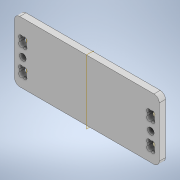
# Autodesk Inventor part: side_side
Saved by Autodesk Inventor 2020 (Build 240168000, 168)
## iProperties
Created: 2020-01-09
Part Number: side_side
Material: Generic
Document SubType Name: Modeling
Designer: erwin
Density: 1 g/cm^3
Appearance: Default
Author: erwin
Autodesk Inventor part; units mm, degrees
ref_plane "YZ Plane" through (0, 0, 0) normal (1, 0, 0) x (0, 1, 0)
ref_plane "XZ Plane" through (0, 0, 0) normal (0, 1, 0) x (-1, 0, 0)
ref_plane "XY Plane" through (0, 0, 0) normal (0, 0, 1) x (1, 0, 0)
ref_plane "Work Plane1" through (0, 0, 0) normal (0, 0, 1) x (1, 0, 0)
ref_plane "Work Plane2" through (0, 0, 0) normal (0, 0, 1) x (1, 0, 0)
sketch "Sketch2" plane through (0, 0, 0) normal (0, 0, 1) x (1, 0, 0)
  line L0 (-3.6, 30) -> (-3.6, 22) projected
  line L1 (70, 0.0472) -> (70, -3.6) projected
  line L2 (73.6, 0.0472) -> (73.6, -3.6) projected
  line L3 (-3.6, 30) -> (73.6, 30)
  line L4 (73.6, 30) -> (73.6, -3.6)
  line L5 (73.6, -3.6) -> (-3.6, -3.6)
  line L6 (-3.6, -3.6) -> (-3.6, 30)
  line L7 (70, 7) -> (70, 2) projected
  line L8 (73.6, 7) -> (73.6, 2) projected
  line L9 (70, 22) -> (70, 17) projected
  line L10 (73.6, 22) -> (73.6, 17) projected
  line L11 (0, 22) -> (-3.6, 22) projected
  line L12 (-3.6, 17) -> (-3.6, 22) projected
  line L13 (-3.6, 17) -> (0, 17) projected
  line L14 (0, 17) -> (0, 22) projected
  line L15 (-3.6, 2) -> (0, 2) projected
  line L16 (0, 2) -> (0, 7) projected
  line L17 (0, 7) -> (-3.6, 7) projected
  line L18 (-3.6, 2) -> (-3.6, 7) projected
  line L19 (70, 2) -> (73.6, 2) projected
  line L20 (70, 7) -> (73.6, 7) projected
  line L21 (70, 17) -> (73.6, 17) projected
  line L22 (70, 22) -> (73.6, 22) projected
  line L23 (70, 0.0472) -> (73.6, 0.0472) projected
  line L24 (70, -3.6) -> (73.6, -3.6) projected
  point P0 (0, 0)
  point P1 (-3.6, 22)
  constraints: 8 end point, 2 parallel, 1 horizontal, 1 perpendicular
extrude "Extrusion1" add sketch "Sketch2" along normal blind 3.6 contours L3 L4 L22 L9 L21 L20 L7 L19 L23 L1 L5 L6 L15 L16 L17 L13 L14 L11 L0 | L1 L23 L2 L5
ref_plane "Work Plane6" through (35, -3.6, 0) normal (1, 0, 0) x (0, 0, -1)
sketch "Sketch3" plane through (0, 0, 3.6) normal (0, 0, 1) x (1, 0, 0)
  line L0 (-3.6, 30) -> (-3.6, 22) projected
  line L1 (73.6, -3.6) -> (73.6, 2) projected
  line L2 (73.6, 30) -> (-3.6, 30) projected
  line L3 (-3.6, 30) -> (-3.6, -3.6) projected
  line L4 (-3.6, 30) -> (-3.6, 30)
  line L5 (-6.6, 27) -> (-6.6, -0.6)
  line L6 (-3.6, -3.6) -> (-3.6, -3.6)
  line L7 (-3.6, -3.6) -> (-3.6, 30)
  arc A0 (-3.6, 30) -> (-6.6, 27) centre (-3.6, 27) ccw
  arc A1 (-6.6, -0.6) -> (-3.6, -3.6) centre (-3.6, -0.6) ccw
  line L8 (-3.6, -3.6) -> (73.6, -3.6) projected
  line L9 (70, 2) -> (70, 7) projected
  line L10 (70, 7) -> (73.6, 7) projected
  line L11 (73.6, 7) -> (73.6, 17) projected
  line L12 (73.6, 17) -> (70, 17) projected
  line L13 (70, 17) -> (70, 22) projected
  line L14 (70, 22) -> (73.6, 22) projected
  line L15 (73.6, 22) -> (73.6, 30) projected
  line L16 (-3.6, 22) -> (0, 22) projected
  line L17 (0, 22) -> (0, 17) projected
  line L18 (0, 17) -> (-3.6, 17) projected
  line L19 (-3.6, 17) -> (-3.6, 7) projected
  line L20 (-3.6, 7) -> (0, 7) projected
  line L21 (0, 7) -> (0, 2) projected
  line L22 (0, 2) -> (-3.6, 2) projected
  line L23 (-3.6, 2) -> (-3.6, -3.6) projected
  line L24 (73.6, 2) -> (70, 2) projected
  point P0 (0, 0)
  point P1 (-6.6, -3.6)
  point P2 (-3.6, 22)
  point P3 (-3.6, 30)
  point P4 (-3.6, 30)
  dimension "d2" = 3
  dimension "d3" = 3
  constraints: 8 end point, 4 point on circle, 4 tangent, 2 centre point, 2 parallel, 2 point on line, 1 equal radius, 1 horizontal, 1 perpendicular
  measures "d2" distance of L3.end point (-6.6, -3.6)
  measures "d3" radius of A0
extrude "Extrusion2" add sketch "Sketch3" against normal blind 3.6 contours L0 L3 A1 L5 A0
sketch "Sketch4" plane through (0, 0, 0) normal (0, 0, -1) x (-1, 0, 0)
  line L0 (0, -3.6) -> (-70, -3.6) projected
  line L1 (0, 0) -> (0, -3.6) projected
  line L2 (-70, 0) -> (0, 0) projected
  line L3 (-70, 0) -> (-70, -3.6) projected
extrude "Extrusion3" cut sketch "Sketch4" against normal blind 1.8
move faces "Move1" translate (0, -0.4, 0) faces at (23.3333, 0, 0.6)
mirror "Mirror3" about plane through (35, -3.6, 0) normal (1, 0, 0) of "Extrusion2"
sketch "Sketch5" plane through (0, 0, 3.6) normal (0, 0, 1) x (1, 0, 0)
  line L0 (0, 17) -> (-3.6, 17) construction
  line L1 (-1.8, 17) -> (-1.8, 7) construction
  line L2 (-3.6, 7) -> (0, 7) construction
  line L3 (73.6, 17) -> (70, 17) construction
  line L4 (71.8, 17) -> (71.8, 7) construction
  line L5 (70, 7) -> (73.6, 7) construction
  point P0 (0, 0)
  point P1 (-1.8, 12)
  point P2 (71.8, 12)
  constraints: 6 midpoint, 4 end point
hole "Hole1" at (-1.8, 12, 3.6) at (71.8, 12, 3.6) direction (0, 0, -1) diameter 3 end through all
sketch "Sketch7" plane through (0, 0, 0) normal (0, 0, -1) x (-1, 0, 0)
  line L0 (-70, 28) -> (-71.8, 28) projected
  line L1 (-71.8, 28) -> (-71.8, 24) projected
  line L2 (-71.8, 24) -> (-70, 24) projected
  line L3 (-70, 30) -> (-70, 28) projected
  line L4 (-73.6, 30) -> (-73.6, 23.9528) projected
  line L5 (-70, 30) -> (-73.6, 30) projected
  line L6 (0, 24) -> (1.8, 24) projected
  line L7 (1.8, 24) -> (1.8, 28) projected
  line L8 (1.8, 28) -> (0, 28) projected
  line L9 (0, 30) -> (0, 28) projected
  line L10 (0, 30) -> (3.6, 30) projected
  line L11 (3.6, 30) -> (3.6, 23.9528) projected
  line L12 (0, 24) -> (0, 23.9528) projected
  line L13 (-71.8, 28) -> (1.8, 28)
  line L14 (1.8, 28) -> (1.8, 24)
  line L15 (1.8, 24) -> (-71.8, 24)
  line L16 (-71.8, 24) -> (-71.8, 28)
  line L17 (3.6, 23.9528) -> (0, 23.9528) projected
  line L18 (-70, 23.9528) -> (-73.6, 23.9528) projected
  line L19 (-70, 24) -> (-70, 23.9528) projected
  point P0 (0, 0)
  constraints: 8 end point, 2 parallel, 1 horizontal, 1 perpendicular
extrude "Extrusion5" cut sketch "Sketch7" against normal blind 1.8 contours L13 L8 L7 L6 L15 L2 L1 L0
sketch "Sketch10" plane through (0, 0, 3.6) normal (0, 0, 1) x (1, 0, 0)
  circle A0 centre (-1.8, 12) radius 1.5 projected
  circle A1 centre (71.8, 12) radius 1.5 projected
  line L0 (73.6, 30) -> (-3.6, 30) projected
  arc A2 (-3.6, 30) -> (-6.6, 27) centre (-3.6, 27) ccw projected
  line L1 (-6.6, 27) -> (-6.6, -0.6) projected
  arc A3 (-6.6, -0.6) -> (-3.6, -3.6) centre (-3.6, -0.6) ccw projected
  line L2 (-3.6, -3.6) -> (73.6, -3.6) projected
  arc A4 (73.6, -3.6) -> (76.6, -0.6) centre (73.6, -0.6) ccw projected
  line L3 (76.6, 27) -> (76.6, -0.6) projected
  arc A5 (76.6, 27) -> (73.6, 30) centre (73.6, 27) ccw projected
  line L4 (73.6, 17) -> (73.6, 22) projected
  line L5 (73.6, 17) -> (70, 17) projected
  line L6 (70, 17) -> (70, 22) projected
  line L7 (70, 22) -> (73.6, 22) projected
  line L8 (73.6, 2) -> (73.6, 7) projected
  line L9 (73.6, 2) -> (70, 2) projected
  line L10 (70, 2) -> (70, 7) projected
  line L11 (70, 7) -> (73.6, 7) projected
  line L12 (-3.6, 2) -> (-3.6, 7) projected
  line L13 (-3.6, 7) -> (0, 7) projected
  line L14 (0, 7) -> (0, 2) projected
  line L15 (0, 2) -> (-3.6, 2) projected
  line L16 (-3.6, 17) -> (-3.6, 22) projected
  line L17 (-3.6, 22) -> (0, 22) projected
  line L18 (0, 22) -> (0, 17) projected
  line L19 (0, 17) -> (-3.6, 17) projected
  line L20 (0.2, 1.8) -> (0.2, 7.2)
  line L21 (0.2, 7.2) -> (-3.8, 7.2)
  line L22 (-3.8, 7.2) -> (-3.8, 1.8)
  line L23 (-3.8, 1.8) -> (0.2, 1.8)
  circle A6 centre (-0.7899, 2.7899) radius 1.4
  line L24 (-1.7799, 1.8) -> (0.2, 1.8) construction
  line L25 (0.2, 1.8) -> (0.2, 3.7799) construction
  line L26 (0.2, 3.7799) -> (-1.7799, 3.7799) construction
  line L27 (-1.7799, 3.7799) -> (-1.7799, 1.8) construction
  line L28 (-1.7799, 1.8) -> (0.2, 3.7799) construction
  line L29 (0.2, 1.8) -> (-1.7799, 3.7799) construction
  circle A7 centre (-0.7899, 6.2101) radius 1.4
  line L30 (-1.7799, 5.2201) -> (0.2, 5.2201) construction
  line L31 (0.2, 5.2201) -> (0.2, 7.2) construction
  line L32 (0.2, 7.2) -> (-1.7799, 7.2) construction
  line L33 (-1.7799, 7.2) -> (-1.7799, 5.2201) construction
  line L34 (-1.7799, 5.2201) -> (0.2, 7.2) construction
  line L35 (0.2, 5.2201) -> (-1.7799, 7.2) construction
  circle A8 centre (-2.8101, 6.2101) radius 1.4
  line L36 (-3.8, 5.2201) -> (-1.8201, 5.2201) construction
  line L37 (-1.8201, 5.2201) -> (-1.8201, 7.2) construction
  line L38 (-1.8201, 7.2) -> (-3.8, 7.2) construction
  line L39 (-3.8, 7.2) -> (-3.8, 5.2201) construction
  line L40 (-3.8, 5.2201) -> (-1.8201, 7.2) construction
  line L41 (-1.8201, 5.2201) -> (-3.8, 7.2) construction
  circle A9 centre (-2.8101, 2.7899) radius 1.4
  line L42 (-3.8, 1.8) -> (-1.8201, 1.8) construction
  line L43 (-1.8201, 1.8) -> (-1.8201, 3.7799) construction
  line L44 (-1.8201, 3.7799) -> (-3.8, 3.7799) construction
  line L45 (-3.8, 3.7799) -> (-3.8, 1.8) construction
  line L46 (-3.8, 1.8) -> (-1.8201, 3.7799) construction
  line L47 (-1.8201, 1.8) -> (-3.8, 3.7799) construction
  line L48 (0, 7) -> (0, 2) projected
  point P0 (0, 0)
  point P1 (0.2, 1.8)
  point P2 (0.2, 3.7799)
  point P3 (0.2, 5.2201)
  point P4 (-1.7799, 7.2)
  point P5 (-1.8, 1.8205)
  point P6 (-1.7799, 1.8)
  point P7 (-1.8201, 1.8)
  point P8 (-3.8, 3.7799)
  point P9 (0.2, 1.8)
  point P10 (-3.8, 5.2201)
  point P11 (-1.8201, 7.2)
  point P12 (0, 2)
  dimension "d34" = 2.8
  dimension "d35" = 2.8
  dimension "d37" = 2.8
  dimension "d39" = 2.8
  dimension "extra_sides_square_holes" = 0.2
  constraints: 56 end point, 8 midpoint, 8 parallel, 8 perpendicular, 4 horizontal, 1 coincident, 15 other
  measures "extra_sides_square_holes" distance between parallel lines of L14 L20
extrude "Extrusion6" cut sketch "Sketch10" against normal through all contours L15 A6 A9 L23 L22 L12 | L12 A9 A6 L15 | A9 L22 A8 L12 | L12 A8 A7 L14 A6 A9 | A6 A9 L15 | L15 A9 A6 | A8 L22 L21 A7 L13 L12 | L12 L13 A7 A8 | A6 L14 L15 A9 | L22 A9 | L15 L14 A6 L20 L23 A9 | A6 L23 A9 | A8 L22 | A8 L13 L14 A7 | A7 L13 A8 | L14 A7 L20 A6 | L23 A9 | L23 A6 | A7 A8 L13 | A8 L21 | L14 L13 A8 A7 L21 L20 | A6 L20 | A8 L21 A7 | L20 A7 | A7 L21
sketch "Sketch11" plane through (0, 0, 3.6) normal (0, 0, 1) x (1, 0, 0)
  line L0 (0, 22) -> (0, 17) projected
  line L1 (73.6, 17) -> (70, 17) projected
  line L2 (73.6, 2) -> (73.6, 7) projected
  point P0 (0, 0)
  point P1 (0, 2)
pattern_sketch "Sketch Driven Pattern1" of "Extrusion6" from (0, 2, 3.6) copies at (0, 17, 3.6) at (73.6, 17, 3.6) at (73.6, 2, 3.6)
thicken "Thicken1" operation add thickness 0.4 both sides no extend neighbours yes toward (0.0804666, -0.9967573, 0) faces at (-1.6793, 10.5049, 2.4)
thicken "Thicken2" operation add thickness 0.4 both sides no extend neighbours yes toward (0.0804666, -0.9967573, 0) faces at (71.9207, 10.5049, 2.4)
thicken "Thicken3" operation add thickness 1 both sides no extend neighbours yes toward (-1, 0, 0) faces at (-1.8, 25.3333, 0.6)
thicken "Thicken4" operation add thickness 1 both sides no extend neighbours yes toward (-1, 0, 0) faces at (0, -2.5333, 0.6)
thicken "Thicken5" operation add thickness 1 both sides no extend neighbours yes toward (1, 0, 0) faces at (71.8, 26.6667, 0.6)
thicken "Thicken6" operation add thickness 1 both sides no extend neighbours yes toward (1, 0, 0) faces at (70, -1.4667, 0.6)
thicken "Thicken7" operation add thickness 0.4 both sides no extend neighbours yes toward (0, 1, 0) faces at (23, -0.4, 0.6)
thicken "Thicken8" operation add thickness 0.2 both sides no extend neighbours yes toward (0, 1, 0) faces at (47.6, 28, 1.2)
thicken "Thicken9" operation add thickness 0.2 both sides no extend neighbours yes toward (0, -1, 0) faces at (47.6, 24, 0.6)
move faces "Move2" translate (0, 1.45, 0) faces at (47.8667, 30, 1.2)
equation "\"d6\" = deep_for_sliding_cover"
equation "\"d11\" = screw_diameter"
equation "\"d20\" = deep_for_sliding_cover"
equation "\"d34\" = bit_diameter"
equation "\"d35\" = d36"
equation "\"d37\" = d38"
equation "\"d39\" = d40"
equation "\"d32\" = extra_for_holes"
equation "\"d33\" = extra_for_holes"
equation "\"d41\" = 0.5 * rails_slack_extra_sides"
equation "\"d42\" = 0.5 * rails_slack_extra_sides"
equation "\"d43\" = 0.5 * rails_slack_extra_sides"
equation "\"d44\" = 0.5 * rails_slack_extra_sides"
equation "\"d45\" = 0.5 * rails_slack_extra_sides"
equation "\"d46\" = 0.5 * rails_slack_extra_sides"
equation "\"d47\" = 0.5 * rails_slack_extra_sides"
equation "\"d48\" = 0.5 * rails_slack_extra_sides"
equation "\"d49\" = rails_slack_extra"
equation "\"d50\" = rails_slack_extra"
equation "\"d51\" = 0.5 * rails_slack_extra"
equation "\"d52\" = 0.5 * rails_slack_extra"
equation "\"d53\" = 0.5 * rails_slack_extra"
equation "\"d54\" = 0.5 * rails_slack_extra"
equation "\"d10\" = extra_for_sliding_cover"
equation "\"deep_for_sliding_cover\" = 1.8"
equation "\"screw_diameter\" = 3"
equation "\"bit_diameter\" = 2.8"
equation "\"d36\" = 2.8"
equation "\"d38\" = 2.8"
equation "\"d40\" = 2.8"
equation "\"extra_for_holes\" = 0.4"
equation "\"rails_slack_extra_sides\" = 2"
equation "\"rails_slack_extra\" = 0.4"
equation "\"extra_for_sliding_cover\" = 0.4"
body "Solid1"
